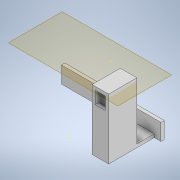
# Autodesk Inventor part: Drehmomentstütze
Saved by Autodesk Inventor 2020 (Build 240168000, 168)
## iProperties
Created: 2019-08-24
Part Number: Drehmomentstütze
Material: Generisch
Document SubType Name: Modeling
Designer: Limmer
Density: 1 g/cm^3
Appearance: Vorgabe
Author: Limmer
Autodesk Inventor part; units mm, degrees
ref_plane "YZ Plane" through (0, 0, 0) normal (1, 0, 0) x (0, 1, 0)
ref_plane "XY Plane" through (0, 0, 0) normal (0, 0, 1) x (1, 0, 0)
sketch "Skizze1" plane through (0, 0, 0) normal (0, 0, 1) x (1, 0, 0)
  line L0 (-60, 0) -> (60, 0)
  line L1 (60, 0) -> (60, 20)
  line L2 (60, 20) -> (-60, 20)
  line L3 (-60, 20) -> (-60, 0)
  point P0 (0, 0)
  dimension "d0" = 120
  dimension "d1" = 20
  constraints: 8 end point, 2 parallel, 1 horizontal, 1 perpendicular
  measures "d0" distance of L2.end L1.end
  measures "d1" distance of L1.end L0.end
extrude "Extrusion1" add sketch "Skizze1" against normal blind 4
sketch "Skizze2" plane through (0, 0, 0) normal (0, 1, 0) x (-1, 0, 0)
  line L0 (-60, 0) -> (60, 0) projected
  line L1 (-52, 0) -> (-32, 0)
  line L2 (-32, 0) -> (-32, 55)
  line L3 (-32, 55) -> (-52, 55)
  line L4 (-52, 55) -> (-52, 0)
  point P0 (0, 0)
  dimension "d17" = 20
  dimension "d18" = 55
  constraints: 8 end point, 2 parallel, 1 horizontal, 1 perpendicular, 1 point on line
  measures "d17" distance of L3.end L2.end
  measures "d18" distance of L2.end L1.end
extrude "Extrusion2" add sketch "Skizze2" along normal blind 4
sketch "Skizze8" plane through (0, 4, 0) normal (0, 1, 0) x (1, 0, 0)
  line L0 (52, -55) -> (52, 0) projected
  line L1 (32, -55) -> (52, -55)
  line L2 (52, -55) -> (52, -51)
  line L3 (52, -51) -> (32, -51)
  line L4 (32, -51) -> (32, -55)
  point P0 (0, 0)
  constraints: 8 end point, 2 parallel, 1 horizontal, 1 perpendicular, 1 point on line
extrude "Extrusion7" add sketch "Skizze8" along normal blind 50
sketch "Skizze9" plane through (0, 4, 0) normal (0, 1, 0) x (1, 0, 0)
  line L0 (32, 0) -> (32, -51) projected
  line L1 (32, -51) -> (36, -51)
  line L2 (36, -51) -> (36, -31)
  line L3 (36, -31) -> (32, -31)
  line L4 (32, -31) -> (32, -51)
  line L5 (52, -51) -> (48, -51)
  line L6 (48, -51) -> (48, -31)
  line L7 (48, -31) -> (52, -31)
  line L8 (52, -31) -> (52, -51)
  point P0 (0, 0)
  constraints: 16 end point, 4 parallel, 2 horizontal, 2 perpendicular, 2 point on line
extrude "Extrusion8" add sketch "Skizze9" along normal blind 65
sketch "Skizze10" plane through (48, 4, 51) normal (0, 0, -1) x (-1, 0, 0)
  point P0 (48, -4)
sketch "Skizze11" plane through (0, 4, 0) normal (0, 1, 0) x (1, 0, 0)
  line L0 (48, -51) -> (36, -51) projected
  line L1 (36, -31) -> (32, -31) projected
  line L2 (48, -51) -> (36, -51)
  line L3 (36, -51) -> (36, -31)
  line L4 (36, -31) -> (48, -31)
  line L5 (48, -31) -> (48, -51)
  point P0 (0, 0)
  constraints: 8 end point, 2 parallel, 1 horizontal, 1 perpendicular
extrude "Extrusion9" add sketch "Skizze11" along normal blind 20
ref_plane "Arbeitsebene1" through (0, 69, 0) normal (0, 1, 0) x (-1, 0, 0)
sketch "Skizze12" plane through (0, 69, 0) normal (0, 1, 0) x (-1, 0, 0)
  line L0 (-32, 0) -> (-32, 55) projected
  line L1 (-52, 55) -> (-32, 55)
  line L2 (-32, 55) -> (-32, 25)
  line L3 (-32, 25) -> (-52, 25)
  line L4 (-52, 25) -> (-52, 55)
  point P0 (0, 0)
  constraints: 8 end point, 2 parallel, 1 horizontal, 1 perpendicular, 1 point on line
extrude "Extrusion10" add sketch "Skizze12" along normal blind 4
sketch "Skizze13" plane through (0, 54, 0) normal (0, 1, 0) x (1, 0, 0)
  point P0 (0, 0)
sketch "Skizze14" plane through (0, 54, 0) normal (0, 1, 0) x (1, 0, 0)
  line L0 (52, -55) -> (52, -25) projected
  line L1 (48, -31) -> (48, -51) projected
  line L2 (52, -55) -> (48, -55)
  line L3 (48, -55) -> (48, -51)
  line L4 (48, -51) -> (52, -51)
  line L5 (52, -51) -> (52, -55)
  line L6 (32, -55) -> (36, -55)
  line L7 (36, -55) -> (36, -51)
  line L8 (36, -51) -> (32, -51)
  line L9 (32, -51) -> (32, -55)
  point P0 (0, 0)
  constraints: 16 end point, 4 parallel, 2 horizontal, 2 perpendicular, 2 point on line
extrude "Extrusion11" add sketch "Skizze14" along normal blind 15
sketch "Skizze15" plane through (0, 69, 0) normal (0, 1, 0) x (-1, 0, 0)
  line L0 (-52, 25) -> (-32, 25) projected
  line L1 (-52, 31) -> (-52, 0) projected
  line L2 (-32, 25) -> (-52, 25)
  line L3 (-52, 25) -> (-52, 21)
  line L4 (-52, 21) -> (-32, 21)
  line L5 (-32, 21) -> (-32, 25)
  point P0 (0, 0)
  constraints: 8 end point, 2 parallel, 1 horizontal, 1 perpendicular, 1 point on line
extrude "Extrusion12" add sketch "Skizze15" along normal blind 4
sketch "Skizze16" plane through (0, 4, 0) normal (0, 1, 0) x (1, 0, 0)
  line L0 (52, -21) -> (32, -21) projected
  line L1 (52, -31) -> (48, -31) projected
  line L2 (52, -21) -> (48, -21)
  line L3 (48, -21) -> (48, -31)
  line L4 (48, -31) -> (52, -31)
  line L5 (52, -31) -> (52, -21)
  line L6 (32, -21) -> (32, -55) projected
  line L7 (36, -31) -> (32, -31) projected
  line L8 (32, -21) -> (36, -21)
  line L9 (36, -21) -> (36, -31)
  line L10 (36, -31) -> (32, -31)
  line L11 (32, -31) -> (32, -21)
  point P0 (0, 0)
  constraints: 16 end point, 4 parallel, 2 horizontal, 2 perpendicular
extrude "Extrusion13" add sketch "Skizze16" along normal blind 65
